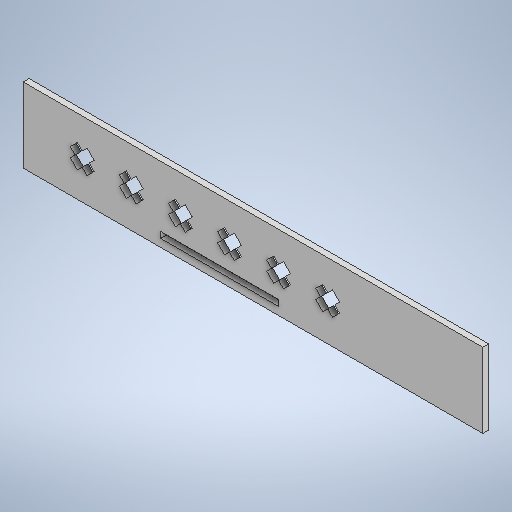
# Autodesk Inventor part: Extension .1
Saved by Autodesk Inventor 2025.4 (Build 294407000, 407)
## iProperties
Created: 2026-06-10
Part Number: Extension .1
Material: Generic
Document SubType Name: Sheet Metal
Designer: lenovo
Density: 1 g/cm^3
Sheet Metal Rule: Default_mm
Appearance: Default
Author: lenovo
Autodesk Inventor part; units mm, degrees
ref_plane "YZ Plane" through (0, 0, 0) normal (1, 0, 0) x (0, 1, 0)
ref_plane "XZ Plane" through (0, 0, 0) normal (0, 1, 0) x (-1, 0, 0)
ref_plane "XY Plane" through (0, 0, 0) normal (0, 0, 1) x (1, 0, 0)
sketch "Sketch1" plane through (0, 0, 0) normal (0, 0, 1) x (1, 0, 0)
  line L0 (-117, -19) -> (117, -19)
  line L1 (117, -19) -> (117, 19)
  line L2 (117, 19) -> (-117, 19)
  line L3 (-117, 19) -> (-117, -19)
  line L4 (-117, -19) -> (117, 19) construction
  line L5 (117, -19) -> (-117, 19) construction
  line L6 (-47.035, -11.93) -> (13.035, -11.93)
  line L7 (13.035, -11.93) -> (13.035, -15)
  line L8 (13.035, -15) -> (-47.035, -15)
  line L9 (-47.035, -15) -> (-47.035, -11.93)
  line L10 (-47.035, -11.93) -> (13.035, -15) construction
  line L11 (13.035, -11.93) -> (-47.035, -15) construction
  point P0 (0, 0)
  point P1 (-17, -13.465)
  dimension "d0" = 38
  dimension "d1" = 234
  dimension "d2" = 100
  dimension "d3" = 3.07
  dimension "d4" = 4
  dimension "d5" = 60.07
  measures "d0" distance between parallel lines of L2 L0
  measures "d1" distance of L1.end L2.end
  measures "d2" distance from line of L3 point (-17, -13.465)
  measures "d3" distance between parallel lines of L6 L8
  measures "d4" distance between parallel lines of L8 L0
  measures "d5" distance of L6.start L6.end
extrude "Plate1" add sketch "Sketch1" along normal blind 3
sketch "Sketch2" plane through (0, 0, 3) normal (0, 0, 1) x (1, 0, 0)
  line L0 (-84.5251, 6.0599) -> (-93.0599, -2.4749)
  line L1 (-93.0599, -2.4749) -> (-89.4749, -6.0599)
  line L2 (-89.4749, -6.0599) -> (-80.9401, 2.4749)
  line L3 (-80.9401, 2.4749) -> (-84.5251, 6.0599)
  line L4 (-89.4749, 6.0599) -> (-93.0599, 2.4749)
  line L5 (-93.0599, 2.4749) -> (-84.5251, -6.0599)
  line L6 (-84.5251, -6.0599) -> (-80.9401, -2.4749)
  line L7 (-80.9401, -2.4749) -> (-89.4749, 6.0599)
  line L8 (-82.7326, 4.2674) -> (-91.2674, -4.2674)
  line L9 (-91.2674, 4.2674) -> (-82.7326, -4.2674)
  line L10 (-117, 19) -> (-117, -19) projected
  line L11 (-117, 0) -> (0, 0)
  line L12 (-117, -19) -> (-117, 19) projected
  point P0 (-87, 0)
  point P1 (-87, -3.585)
  point P2 (-83.415, 0)
  point P3 (-87, 3.585)
  point P4 (-90.585, 0)
  dimension "d7" = 5.07
  dimension "d8" = 30
  dimension "d9" = 12.07
  dimension "d11" = 45
  constraints: 22 end point, 8 midpoint, 5 perpendicular, 4 parallel, 1 horizontal, 1 point on line
  measures "d7" distance of L4.start L4.end
  measures "d8" distance of point (-117, 0) point (-87, 0)
  measures "d9" distance of L6.end L4.start
  measures "d11" angle of L9 L11
extrude "Cut1" cut sketch "Sketch2" against normal blind 3
pattern_linear "Rectangular Pattern1" count 6 spacing 25 along (1, 0, 0) of "Cut1"
equation "\"d12\" = Thickness"
equation "\"d6\" = Thickness"
equation "\"BendRadius\" = Thickness"
equation "\"BendReliefWidth\" = Thickness"
equation "\"BendReliefDepth\" = 0.5 * Thickness"
equation "\"CornerReliefSize\" = 4 * Thickness"
equation "\"MinimumRemnant\" = 2 * Thickness"
equation "\"TransitionRadius\" = BendRadius"
equation "\"JacobiRadiusSize\" = BendRadius"
equation "\"GapSize\" = Thickness"
equation "\"Thickness\" = 3"
body "Solid1"
